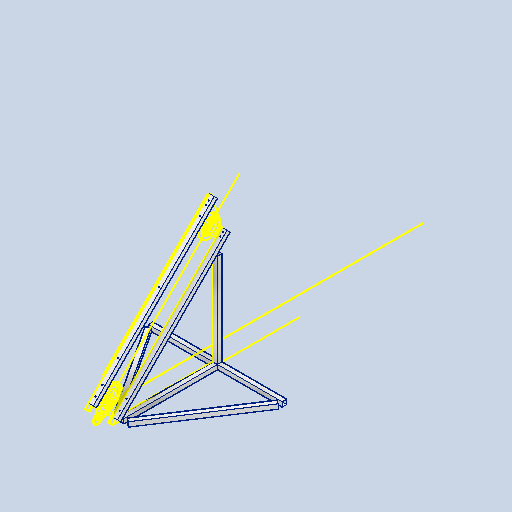
# Autodesk Inventor part: belt_liner_v1_ASP_Base
Saved by Autodesk Inventor 2025.1 (Build 291241000, 241)
## iProperties
Created: 2024-12-08
Part Number: belt_liner_v1_ASP_Base
Material: アルミニウム 6061
Document SubType Name: Modeling
Designer: haruy
Density: 2.7 g/cm^3
Appearance: アルミニウム - フラット
Author: haruy
Autodesk Inventor part; units mm, degrees
ref_plane "YZ Plane" through (0, 0, 0) normal (1, 0, 0) x (0, 1, 0)
ref_plane "XZ Plane" through (0, 0, 0) normal (0, 1, 0) x (-1, 0, 0)
ref_plane "XY Plane" through (0, 0, 0) normal (0, 0, 1) x (1, 0, 0)
derived "belt_liner_v1_Sketch_Base.ipt"
sketch "スケッチ1" plane through (300, 0, 0) normal (1, 0, 0) x (0, 1, 0)
  circle A0 centre (0, 0) radius 23.875
  circle A1 centre (323.28922, -323.28922) radius 23.875
  line L0 (0, 0) -> (0, -985.832038)
  line L1 (14.142136, 50.310647) -> (24.748737, 60.917249)
  line L2 (24.748737, 60.917249) -> (406.586399, -320.920413)
  line L3 (406.586399, -320.920413) -> (395.979797, -331.527014)
  line L4 (395.979797, -331.527014) -> (14.142136, 50.310647)
  line L5 (0, 0) -> (323.28922, -323.28922)
  line L6 (-50.310647, -14.142136) -> (-60.917249, -24.748737)
  line L7 (-60.917249, -24.748737) -> (289.100607, -374.766594)
  line L8 (289.100607, -374.766594) -> (299.707209, -364.159992)
  line L9 (299.707209, -364.159992) -> (-50.310647, -14.142136)
  line L10 (22.552369, 63.113618) -> (22.552369, 63.113618)
  line L11 (14.142136, 50.310647) -> (71.310915, -6.858132)
  line L12 (71.310915, -6.858132) -> (67.775381, -10.393666)
  line L13 (67.775381, -10.393666) -> (10.606602, 46.775114)
  line L14 (10.606602, 46.775114) -> (14.142136, 50.310647)
  line L15 (395.979797, -331.527014) -> (376.534361, -312.081578)
  line L16 (376.534361, -312.081578) -> (372.998827, -315.617112)
  line L17 (372.998827, -315.617112) -> (392.444264, -335.062548)
  line L18 (392.444264, -335.062548) -> (395.979797, -331.527014)
  line L19 (0, -985.832038) -> (0, 0)
  circle A2 centre (0, 0) radius 12.5
  circle A3 centre (21.213203, -21.213203) radius 23.5
  circle A4 centre (0, 0) radius 15
  circle A5 centre (21.213203, -21.213203) radius 15
  line L20 (0, 0) -> (0, 0)
  circle A6 centre (-21.213203, 21.213203) radius 15
  circle A7 centre (-21.213203, 21.213203) radius 12.25
  circle A8 centre (0, 0) radius 25.575
  line L21 (0, 0) -> (0, 0)
  line L22 (0, 0) -> (0, 0)
  circle A9 centre (52.713203, -21.213203) radius 1.5
  circle A10 centre (21.213203, -21.213203) radius 31.5
  line L23 (21.213203, -21.213203) -> (49.904061, 7.477654)
  circle A11 centre (21.213203, 10.286797) radius 1.5
  circle A12 centre (-10.286797, -21.213203) radius 1.5
  circle A13 centre (21.213203, -52.713203) radius 1.5
  circle A14 centre (21.213203, -52.713203) radius 3
  circle A15 centre (52.713203, -21.213203) radius 3
  circle A16 centre (21.213203, -52.713203) radius 3
  circle A17 centre (-10.286797, -21.213203) radius 3
  circle A18 centre (21.213203, 10.286797) radius 3
  line L24 (23.334524, 12.408117) -> (54.834524, -19.091883)
  line L25 (54.834524, -23.334524) -> (23.334524, -54.834524)
  line L26 (19.091883, -54.834524) -> (-12.408117, -23.334524)
  line L27 (-50.310647, -14.142136) -> (-46.775114, -10.606602)
  line L28 (-46.775114, -10.606602) -> (10.393666, -67.775381)
  line L29 (10.393666, -67.775381) -> (6.858132, -71.310915)
  line L30 (6.858132, -71.310915) -> (-50.310647, -14.142136)
  line L31 (-15.722251, 32.163635) -> (22.557926, 12.968535)
  line L32 (-32.163635, 15.722251) -> (-12.968535, -22.557926)
  line L33 (84.852814, 0.813173) -> (406.586399, -320.920413)
  line L34 (406.586399, -320.920413) -> (410.475486, -317.031325)
  line L35 (410.475486, -317.031325) -> (88.741901, 4.70226)
  line L36 (88.741901, 4.70226) -> (84.852814, 0.813173)
  circle A19 centre (323.28922, -323.28922) radius 5
  line L37 (299.707209, -364.159992) -> (280.96888, -345.421663)
  line L38 (280.96888, -345.421663) -> (284.504413, -341.886129)
  line L39 (284.504413, -341.886129) -> (303.242743, -360.624458)
  line L40 (303.242743, -360.624458) -> (299.707209, -364.159992)
  circle A20 centre (319.753686, -319.753686) radius 5
  line L41 (323.28922, -323.28922) -> (417.261527, -417.261527)
  circle A21 centre (337.431356, -337.431356) radius 5
  line L42 (323.28922, -316.218153) -> (340.96689, -333.895822)
  line L43 (316.218153, -323.28922) -> (333.895822, -340.96689)
  circle A22 centre (323.28922, -323.28922) radius 22.175
  circle A23 centre (323.28922, -323.28922) radius 33.875
  line L44 (365.827862, -301.375079) -> (355.22126, -311.981681)
  line L45 (355.22126, -311.981681) -> (358.756794, -315.517214)
  line L46 (358.756794, -315.517214) -> (369.363396, -304.910613)
  line L47 (369.363396, -304.910613) -> (365.827862, -301.375079)
  circle A24 centre (319.753686, -319.753686) radius 10
  circle A25 centre (337.431356, -337.431356) radius 10
  line L48 (326.824754, -312.682619) -> (344.502424, -330.360288)
  line L49 (312.682619, -326.824754) -> (330.360288, -344.502424)
  line L50 (326.824754, -312.682619) -> (318.28922, -304.147085)
  line L51 (312.682619, -312.682619) -> (319.753686, -305.611551)
  line L52 (319.753686, -305.611551) -> (376.534361, -312.081578)
  line L53 (392.444264, -335.062548) -> (303.242743, -360.624458)
  line L54 (344.502424, -330.360288) -> (351.298151, -337.156016)
  line L55 (351.298151, -337.156016) -> (351.573492, -337.431356)
  line L56 (71.310915, -6.858132) -> (67.775381, -10.393666)
  line L57 (67.775381, -10.393666) -> (90.863221, -33.481506)
  line L58 (90.863221, -33.481506) -> (94.398755, -29.945972)
  line L59 (94.398755, -29.945972) -> (71.310915, -6.858132)
  line L60 (244.082751, -334.748737) -> (-45.917249, -334.748737)
  line L61 (-45.917249, -334.748737) -> (-45.917249, -349.748737)
  line L62 (-45.917249, -349.748737) -> (244.082751, -349.748737)
  line L63 (244.082751, -349.748737) -> (244.082751, -334.748737)
  line L64 (-60.917249, -24.748737) -> (-60.917249, -604.283452)
  line L65 (-45.917249, -334.748737) -> (-60.917249, -334.748737)
  line L66 (-60.917249, -334.748737) -> (-60.917249, -349.748737)
  line L67 (-60.917249, -349.748737) -> (-45.917249, -349.748737)
  line L68 (-45.917249, -349.748737) -> (-45.917249, -334.748737)
  line L69 (-60.917249, -334.748737) -> (-45.917249, -334.748737)
  line L70 (-45.917249, -334.748737) -> (-45.917249, -44.748737)
  line L71 (-45.917249, -44.748737) -> (-60.917249, -44.748737)
  line L72 (-60.917249, -44.748737) -> (-60.917249, -334.748737)
  line L73 (330.360288, -344.502424) -> (344.502424, -330.360288)
  line L74 (344.502424, -330.360288) -> (351.573492, -337.431356)
  line L75 (351.573492, -337.431356) -> (337.431356, -351.573492)
  line L76 (337.431356, -351.573492) -> (330.360288, -344.502424)
  line L77 (406.586399, -320.920413) -> (395.979797, -331.527014)
  line L78 (395.979797, -331.527014) -> (399.515331, -335.062548)
  line L79 (399.515331, -335.062548) -> (410.121933, -324.455947)
  line L80 (410.121933, -324.455947) -> (406.586399, -320.920413)
  line L81 (-12.19037, 2.764939) -> (-50.310647, -35.355339)
  line L82 (-12.19037, 2.764939) -> (35.355339, 50.310647)
  line L83 (6.858132, -71.310915) -> (-3.748469, -81.917517)
  line L84 (-22.026376, -35.355339) -> (-36.168512, -49.497475)
  line L85 (-0.813173, -56.568542) -> (-14.955308, -70.710678)
  circle A26 centre (-30.865211, -30.052038) radius 1.5
  circle A27 centre (-13.187541, -47.729708) radius 1.5
  circle A28 centre (2.722361, -63.63961) radius 1.5
  line L86 (49.497475, 36.168512) -> (35.355339, 22.026376)
  line L87 (70.710678, 14.955308) -> (56.568542, 0.813173)
  circle A29 centre (30.052038, 30.865211) radius 1.5
  circle A30 centre (47.729708, 13.187541) radius 1.5
  circle A31 centre (63.63961, -2.722361) radius 1.5
  line L88 (289.454161, -346.835876) -> (285.918627, -350.37141)
  line L89 (297.939442, -355.321158) -> (294.403908, -358.856691)
  circle A32 centre (287.686394, -348.603643) radius 1.5
  circle A33 centre (296.171675, -357.088924) radius 1.5
  line L90 (381.484108, -317.031325) -> (377.948575, -320.566859)
  line L91 (389.96939, -325.516607) -> (386.433856, -329.052141)
  circle A34 centre (379.716341, -318.799092) radius 1.5
  circle A35 centre (388.201623, -327.284374) radius 1.5
  line L92 (284.504413, -341.886129) -> (312.557146, -312.810358)
  line L93 (312.682619, -326.824754) -> (305.614931, -320.005745)
  circle A36 centre (333.895822, -323.28922) radius 1.5
  circle A37 centre (323.28922, -333.895822) radius 1.5
  point P0 (318.28922, -304.147085)
  point P1 (-53.417249, -334.748737)
  point P2 (-45.917249, -334.748737)
  point P3 (-39.704046, -24.748737)
  point P4 (24.748737, 39.704046)
  point P5 (35.355339, 50.310647)
  point P6 (287.686394, -348.603643)
sketch "スケッチ2" plane through (0, 0, 300) normal (0, 0, 1) x (1, 0, 0)
  circle A0 centre (0, 0) radius 120
  circle A1 centre (-88.388348, -88.388348) radius 5
  circle A2 centre (88.388348, -88.388348) radius 5
  line L0 (0, 0) -> (0, -186.303883)
  line L1 (-10, 30) -> (10, 30)
  line L2 (10, 30) -> (10, -30)
  line L3 (10, -30) -> (-10, -30)
  line L4 (-10, -30) -> (-10, 30)
  line L5 (12, 2.5) -> (17, 2.5)
  line L6 (17, 2.5) -> (17, -2.5)
  line L7 (17, -2.5) -> (12, -2.5)
  line L8 (12, -2.5) -> (12, 2.5)
ref_plane "作業平面1" through (300, 0, 0) normal (1, 0, 0) x (0, 1, 0)
ref_plane "作業平面2" through (0, 0, 300) normal (0, 0, 1) x (1, 0, 0)
extrude "押し出し1" add sketch "スケッチ1" along normal blind 15 contours L65 L64 L71 L70
extrude "押し出し2" add sketch "スケッチ1" along normal blind 15 separate body contours L9 L83 L0 | L0 L83 L7 L85 L9 | L9 L8 L7 L0 L83 | L0 L7 L83 | L85 L7 L84 L9 | L81 L7 L6 L9 | L9 L84 L7 L81
extrude "押し出し3" add sketch "スケッチ1" along normal blind 15 separate body contours L60 L63 L62 L0 | L0 L62 L61 L60
shell "シェル1" thickness 1 removed faces 6 at (305, 292.636141, -371.23106) at (305, -53.846181, -17.67767) at (305, -50.917249, -44.748737) at (305, -55.917249, -334.748737) at (305, -45.917249, -339.748737) at (305, 244.082751, -344.748737) bodies 2 1 3
sketch "スケッチ3" plane through (300, -60.917249, -334.748737) normal (0, -1, 0) x (1, 0, 0)
  line L0 (-200, -15) -> (215, -15)
  line L1 (215, -15) -> (215, 0)
  line L2 (215, 0) -> (-200, 0)
  line L3 (-200, 0) -> (-200, -15)
  line L4 (0, 0) -> (15, 0)
  line L5 (-186.830163, 3) -> (-3, 283.056193)
  line L6 (-3, 283.056193) -> (-15.53983, 291.287394)
  line L7 (-15.53983, 291.287394) -> (-199.369992, 11.231201)
  line L8 (-199.369992, 11.231201) -> (-186.830163, 3)
  line L9 (0, 764.698485) -> (0, -144.949747)
  line L10 (15, 290) -> (15, 0)
  line L11 (7.5, 0) -> (7.5, 290)
  line L12 (0, 290) -> (15, 290)
  line L13 (201.830163, 3) -> (18, 283.056193)
  line L14 (18, 283.056193) -> (30.53983, 291.287394)
  line L15 (30.53983, 291.287394) -> (214.369992, 11.231201)
  line L16 (214.369992, 11.231201) -> (201.830163, 3)
  point P0 (-300, 334.748737)
  dimension "d8" = 15
  dimension "d9" = 0
  dimension "d10" = 15
  dimension "d11" = 200
  dimension "d12" = 200
  dimension "d13" = 57.639
  dimension "d14" = 335
  dimension "d15" = 3
  dimension "d16" = 3
  constraints: 26 end point, 4 parallel, 4 symmetric about line, 2 midpoint, 2 perpendicular, 1 horizontal
  measures "d8" distance of L1.end L0.end
  measures "d9" distance between parallel lines of L4 L2
  measures "d10" distance of L6.end L5.end
  measures "d11" distance between parallel lines of L3 L9
  measures "d12" distance between parallel lines of L10 L1
  measures "d14" distance between parallel lines of L8 L6
  measures "d15" distance from line of L5.start L2
  measures "d16" distance from line of L9 L5.end
extrude "押し出し4" add sketch "スケッチ3" against normal blind 15 separate body contours L3 L2 L9 L0 | L9 L2 L1 L0
extrude "押し出し5" add sketch "スケッチ3" against normal blind 15 separate body contours L8 L7 L6 L5 | L13 L14 L15 L16
shell "シェル2" thickness 1 removed faces 6 at (515, -55.917249, -344.748737) at (506.010106, -55.917249, -329.005004) at (326.359886, -55.917249, -46.205077) at (292.820057, -55.917249, -48.94881) at (100, -50.917249, -339.748737) at (104.809951, -55.917249, -326.26127) bodies 4 5
extrude "押し出し6" add sketch "スケッチ1" along normal blind 15 separate body contours L87 L2 L3 L4 | L4 L86 L2 L87 | L4 L82 L2 L86 | L4 L1 L2 L82 | L80 L79 L78 L3
sketch "スケッチ5" plane through (300, 24.748737, 60.917249) normal (0, 0.7071068, 0.7071068) x (1, 0, 0)
  line L0 (0, 0) -> (15, 0) projected
  line L1 (0, 540) -> (0, 0) projected
  point P0 (-300, 25.575)
  point P1 (7.5, 92.5)
  point P2 (7.5, 112.5)
  point P3 (7.5, 132.5)
  point P4 (7.5, 152.5)
  point P5 (7.5, 172.5)
  point P6 (7.5, 192.5)
  point P7 (7.5, 212.5)
  point P8 (7.5, 232.5)
  point P9 (7.5, 252.5)
  point P10 (7.5, 272.5)
  point P11 (7.5, 292.5)
  point P12 (7.5, 312.5)
  point P13 (7.5, 332.5)
  point P14 (7.5, 352.5)
  point P15 (7.5, 372.5)
  point P16 (7.5, 392.5)
  point P17 (7.5, 412.5)
  point P18 (7.5, 432.5)
  point P19 (7.5, 452.5)
  point P20 (7.5, 472.5)
  point P21 (7.5, 492.5)
  point P22 (7.5, 512.5)
  point P23 (7.5, 532.5)
  dimension "d25" = 92.5
  dimension "d26" = 7.5
  dimension "d30" = 20
  constraints: 1 vertical, 22 other
  measures "d25" distance from line of point (7.5, 92.5) L0
  measures "d26" distance from line of L1 point (7.5, 92.5)
  measures "d30" distance of point (7.5, 92.5) point (7.5, 112.5)
shell "シェル4" thickness 1 removed faces 2 at (305, 403.050865, -331.527014) at (310, 21.213203, 57.381715) bodies 6
hole "穴1" at (307.5, 118.440386, -32.774399) at (307.5, 372.998827, -287.332841) at (307.5, 245.719606, -160.05362) direction (0, -0.7071068, -0.7071068) diameter 3.4 end through all bodies 6
extrude "押し出し7" cut sketch "スケッチ1" along normal blind 15 contours L81 L7 L6 L9 bodies 2
extrude "押し出し8" cut sketch "スケッチ1" along normal blind 15 contours L4 L1 L2 L82 bodies 6
sketch "スケッチ6" plane through (300, 299.707209, -364.159992) normal (0, 0.7071068, 0.7071068) x (1, 0, 0)
  line L0 (0, -480) -> (15, -480) projected
  line L1 (15, 0) -> (15, -480) projected
  point P0 (-300, -469.425)
  point P1 (7.5, -460)
  point P2 (7.5, -430)
  point P3 (7.5, -19.5)
  point P4 (7.5, -7.5)
  dimension "d47" = 20
  dimension "d48" = 30
  dimension "d49" = 7.5
  dimension "d50" = 7.5
  dimension "d73" = 410.5
  dimension "d74" = 12
  dimension "d75" = 7.5
  dimension "d76" = 7.5
  measures "d47" distance from line of point (7.5, -460) L0
  measures "d48" distance of point (7.5, -430) point (7.5, -460)
  measures "d49" distance from line of point (7.5, -460) L1
  measures "d50" distance from line of point (7.5, -430) L1
  measures "d73" distance of point (7.5, -430) point (7.5, -19.5)
  measures "d74" distance of point (7.5, -7.5) point (7.5, -19.5)
  measures "d75" distance from line of point (7.5, -19.5) L1
  measures "d76" distance from line of L1 point (7.5, -7.5)
hole "穴2" at (307.5, -25.56191, -38.890873) at (307.5, -4.348707, -60.104076) at (307.5, 285.918627, -350.37141) at (307.5, 294.403908, -358.856691) direction (0, -0.7071068, -0.7071068) diameter 3.4 end through all bodies 2
sketch "スケッチ7" plane through (300, 410.121933, -324.455947) normal (0, 0.7071068, 0.7071068) x (1, 0, 0)
  line L0 (0, -530) -> (15, -530) projected
  line L1 (15, 0) -> (15, -530) projected
  line L2 (0, 0) -> (0, -530) projected
  point P0 (-300, -519.425)
  point P1 (7.5, -510)
  point P2 (7.5, -480)
  point P3 (7.5, -25.5)
  point P4 (7.5, -13.5)
  dimension "d58" = 20
  dimension "d59" = 30
  dimension "d60" = 7.5
  dimension "d61" = 7.5
  dimension "d69" = 12
  dimension "d70" = 7.5
  dimension "d71" = 7.5
  dimension "d72" = 454.5
  measures "d58" distance from line of point (7.5, -510) L0
  measures "d59" distance of point (7.5, -480) point (7.5, -510)
  measures "d60" distance from line of point (7.5, -510) L1
  measures "d61" distance from line of point (7.5, -480) L1
  measures "d69" distance of point (7.5, -25.5) point (7.5, -13.5)
  measures "d70" distance from line of point (7.5, -13.5) L2
  measures "d71" distance from line of point (7.5, -25.5) L2
  measures "d72" distance of point (7.5, -480) point (7.5, -25.5)
hole "穴3" at (307.5, 49.497475, 36.168512) at (307.5, 70.710678, 14.955308) at (307.5, 392.09071, -306.424724) at (307.5, 400.575992, -314.910005) direction (0, -0.7071068, -0.7071068) diameter 3.4 end through all bodies 6
equation "\"d50\" = d49"
equation "\"d76\" = d75"
equation "\"d61\" = d60"
equation "\"d71\" = d70"
